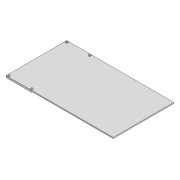
# Autodesk Inventor part: форточка
Saved by Autodesk Inventor 2021 (Build 250183000, 183)
## iProperties
Created: 2023-02-20
Part Number: форточка
Material: Типовые
Document SubType Name: Modeling
Designer: Tasya
Density: 1 g/cm^3
Appearance: По умолчанию
Author: Tasya
Autodesk Inventor part; units mm, degrees
ref_plane "YZ Plane" through (0, 0, 0) normal (1, 0, 0) x (0, 1, 0)
ref_plane "XZ Plane" through (0, 0, 0) normal (0, 1, 0) x (-1, 0, 0)
ref_plane "XY Plane" through (0, 0, 0) normal (0, 0, 1) x (1, 0, 0)
sketch "Эскиз1" plane through (0, 0, 0) normal (0, 1, 0) x (-1, 0, 0)
  line L0 (-150, 85) -> (150, 85)
  line L1 (150, 85) -> (150, -85)
  line L2 (150, -85) -> (-150, -85)
  line L3 (-150, -85) -> (-150, 85)
  line L4 (-150, 85) -> (150, -85) construction
  line L5 (150, 85) -> (-150, -85) construction
  point P0 (0, 0)
  dimension "d0" = 170
  dimension "d1" = 300
  constraints: 12 end point, 2 midpoint, 2 parallel, 1 horizontal, 1 perpendicular
  measures "d0" distance of L0.end L1.end
  measures "d1" distance of L1.end L2.end
extrude "Выдавливание1" add sketch "Эскиз1" along normal blind 3
sketch "Эскиз4" plane through (0, 0, 0) normal (0, -1, 0) x (1, 0, 0)
  line L0 (150, -85) -> (-150, -85) projected
  line L1 (150, 85) -> (150, -85) projected
  line L2 (-150, 85) -> (150, 85) projected
  line L3 (-150, -85) -> (-150, 85) projected
  line L4 (150, -85) -> (-150, -85) projected
  line L5 (-150, -85) -> (-150, 85)
  line L6 (-150, 85) -> (-78, 85)
  line L7 (-78, 85) -> (-78, -85)
  line L8 (-78, -85) -> (-150, -85)
  point P0 (0, 0)
  point P1 (-78, -85)
  point P2 (-78, 85)
  dimension "d17" = 72
  constraints: 8 end point, 2 parallel, 2 perpendicular
  measures "d17" distance between parallel lines of L3 L7
extrude "Выдавливание3" add sketch "Эскиз4" along normal blind 2 contours L0 L3 L2 L7
sketch "Эскиз2" plane through (0, 3, 0) normal (0, 1, 0) x (1, 0, 0)
  line L0 (-82, 81) -> (-146, 81) construction
  line L1 (-146, 81) -> (-146, -81) construction
  line L2 (-146, -81) -> (-82, -81) construction
  line L3 (-82, -81) -> (-82, 81) construction
  line L4 (-82, 81) -> (-146, -81) construction
  line L5 (-146, 81) -> (-82, -81) construction
  line L6 (0, 0) -> (-69.8255, 0) construction
  line L7 (-150, 85) -> (-150, -85) construction
  point P0 (-114, 0)
  point P1 (-114, 0)
  dimension "d4" = 162
  dimension "d5" = 4
  dimension "d6" = 64
  constraints: 14 end point, 4 coincident, 3 midpoint, 2 horizontal, 2 parallel, 1 perpendicular, 1 point on line
  measures "d4" distance of L0.end L1.end
  measures "d5" distance between parallel lines of L7 L1
  measures "d6" distance between parallel lines of L1 L3
hole "Отверстие1" at (-146, 3, 81) at (-82, 3, 81) at (-146, 3, -81) at (-82, 3, -81) direction (0, -1, 0) diameter 3.4 depth 3.7 countersink diameter 6.6 countersink angle 90 clearance for "с потайной головкой ГОСТ 12876-67" size "M3" standard "ГОСТ"
fillet "Сопряжение1" radius 0.5 2 edges at (-78, 0, 0) (-78, -2, 0)
